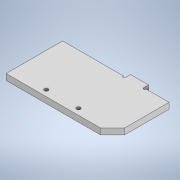
# Autodesk Inventor part: Trunk_lower_flank_frame_
Saved by Autodesk Inventor 2020.4 (Build 244396000, 396)
## iProperties
Created: 2022-01-02
Part Number: Trunk_lower_flank_frame_
Material: 一般
Document SubType Name: Modeling
Designer: Masato Kubotera
Density: 1 g/cm^3
Appearance: 既定
Author: Masato Kubotera
Autodesk Inventor part; units mm, degrees
ref_plane "YZ Plane" through (0, 0, 0) normal (1, 0, 0) x (0, 1, 0)
ref_plane "XZ Plane" through (0, 0, 0) normal (0, 1, 0) x (-1, 0, 0)
ref_plane "XY Plane" through (0, 0, 0) normal (0, 0, 1) x (1, 0, 0)
derived "Trunk_basis.ipt"
sketch "スケッチ1" plane through (0, 0, 0) normal (0, 1, 0) x (-1, 0, 0)
  line L0 (0, 24.5) -> (0, -139) construction
  circle A0 centre (5, 0) radius 10.5 construction
  line L1 (-7, 16) -> (36, 16) construction
  line L2 (36, 16) -> (36, -16) construction
  line L3 (36, -16) -> (-7, -16) construction
  line L4 (-7, -16) -> (-7, 16) construction
  line L5 (-7, 16) -> (36, -16) construction
  line L6 (36, 16) -> (-7, -16) construction
  line L7 (33, 13.5) -> (6, 13.5) construction
  line L8 (6, 13.5) -> (6, -13.5) construction
  line L9 (6, -13.5) -> (33, -13.5) construction
  line L10 (33, -13.5) -> (33, 13.5) construction
  line L11 (33, 13.5) -> (6, -13.5) construction
  line L12 (6, 13.5) -> (33, -13.5) construction
  line L13 (-7, 0) -> (36, 0) construction
  arc A1 (5, 16) -> (-7, 10.583) centre (5, 0) ccw construction
  line L14 (34.5651, -16.05) -> (5, -16.05)
  line L15 (5, 16.05) -> (34.5651, 16.05)
  line L16 (36.05, 14.5651) -> (36.05, -14.5651)
  line L17 (36.05, -16.05) -> (-7.05, 16.05) construction
  line L18 (-7.05, -16.05) -> (36.05, 16.05) construction
  arc A2 (5, 16.05) -> (-6.5314, 11.1638) centre (5, 0) ccw
  arc A3 (-6.5314, 11.1638) -> (-7.05, 9.8372) centre (-6.0721, 10.2196) ccw
  arc A4 (36.05, 14.5651) -> (34.5651, 16.05) centre (35.3075, 15.3075) ccw
  circle A5 centre (6, 13.5) radius 1.35 construction
  line L19 (19.5, 13.5) -> (19.5, -13.5) construction
  circle A6 centre (33, 13.5) radius 1.35 construction
  line L20 (-9.5, 24.5) -> (-14.5, 19.5)
  line L21 (-14.5, 19.5) -> (-14.5, -2.8299)
  line L22 (-14.5, -2.8299) -> (-28.5, -16.8299)
  line L23 (-28.5, -16.8299) -> (-28.5, -94.5)
  line L24 (86.5, -94.5) -> (86.5, -38.5827)
  line L25 (86.5, -38.5827) -> (52.05, -18.693)
  line L26 (52.05, -18.693) -> (52.05, 19.5)
  line L27 (52.05, 19.5) -> (47.05, 24.5)
  line L28 (47.05, 24.5) -> (-9.5, 24.5)
  line L29 (-18.5, -92) -> (-28.5, -102)
  line L30 (-28.5, -102) -> (-28.5, -139)
  line L31 (-28.5, -139) -> (60, -139)
  line L32 (60, -139) -> (60, -92)
  line L33 (60, -92) -> (-18.5, -92)
  line L34 (-16, -139) -> (-16, -99.5) construction
  line L35 (-16, -99.5) -> (16, -99.5) construction
  line L36 (16, -139) -> (16, -99.5) construction
  line L37 (-7.5, -139) -> (-7.5, -143)
  line L38 (-7.5, -143) -> (7.5, -143)
  line L39 (7.5, -139) -> (7.5, -143)
  arc A7 (-7.5, -139) -> (-9.6, -139) centre (-8.55, -139) ccw
  arc A8 (9.6, -139) -> (7.5, -139) centre (8.55, -139) ccw
  line L40 (-20, -139) -> (-20, -133) construction
  line L41 (-21.5, -133) -> (-18.5, -133) construction
  line L42 (-21.5, -133) -> (-21.5, -139) construction
  line L43 (-18.5, -133) -> (-18.5, -139) construction
  line L44 (-12, 22) -> (-7, 22) construction
  line L45 (-7, 22) -> (-7, -22) construction
  line L46 (-7, -22) -> (-12, -22) construction
  line L47 (-12, -22) -> (-12, 22) construction
  line L48 (-12, 22) -> (-7, -22) construction
  line L49 (-7, 22) -> (-12, -22) construction
  line L50 (-9.5, 22) -> (-9.5, -22) construction
  line L51 (-7, 0) -> (-12, 0) construction
  circle A9 centre (-9.5, 17.75) radius 1.6
  line L52 (-12, 10) -> (-9.5, 10) construction
  line L53 (-9.5, 10) -> (-9.5, -10) construction
  line L54 (-9.5, -10) -> (-12, -10) construction
  line L55 (-12, -10) -> (-12, 10) construction
  line L56 (-12, 10) -> (-9.5, -10) construction
  line L57 (-9.5, 10) -> (-12, -10) construction
  line L58 (-9.45, 10.05) -> (-12.05, 10.05)
  line L59 (-12.05, 7.95) -> (-12.05, -7.95)
  line L60 (-12.05, -10.05) -> (-9.45, -10.05)
  line L61 (-9.45, -7.95) -> (-9.45, 7.95)
  line L62 (-9.45, 10.05) -> (-12.05, -10.05) construction
  line L63 (-12.05, 10.05) -> (-9.45, -10.05) construction
  arc A10 (-12.05, 10.05) -> (-12.05, 7.95) centre (-12.05, 9) ccw
  line L64 (-10.75, 10) -> (-10.75, -10) construction
  arc A11 (-9.45, 7.95) -> (-9.45, 10.05) centre (-9.45, 9) ccw
  circle A12 centre (-9.5, -17.75) radius 1.6
  arc A13 (-12.05, -7.95) -> (-12.05, -10.05) centre (-12.05, -9) ccw
  arc A14 (-9.45, -10.05) -> (-9.45, -7.95) centre (-9.45, -9) ccw
  line L65 (36.05, 14.4) -> (44.55, 14.4) construction
  line L66 (44.55, 14.4) -> (44.55, -14.4) construction
  line L67 (36.05, -14.4) -> (44.55, -14.4) construction
  line L68 (44.5, 7.95) -> (44.5, -7.95)
  line L69 (49.55, 0) -> (44.55, 0) construction
  line L70 (44.55, 22) -> (49.55, 22) construction
  line L71 (47.1, -7.95) -> (47.1, 7.95)
  line L72 (45.8, 10) -> (45.8, -10) construction
  line L73 (47.05, 10) -> (44.55, -10) construction
  line L74 (47.05, -10) -> (44.55, -10) construction
  line L75 (47.05, 10) -> (47.05, -10) construction
  line L76 (44.55, 10) -> (47.05, -10) construction
  line L77 (44.5, -10.05) -> (47.1, -10.05)
  line L78 (44.5, 10.05) -> (47.1, -10.05) construction
  line L79 (47.1, 10.05) -> (44.5, -10.05) construction
  line L80 (49.55, -22) -> (44.55, -22) construction
  line L81 (44.55, 22) -> (49.55, -22) construction
  line L82 (49.55, 22) -> (49.55, -22) construction
  line L83 (49.55, 22) -> (44.55, -22) construction
  line L84 (47.05, 22) -> (47.05, -22) construction
  line L85 (44.55, -22) -> (44.55, 22) construction
  circle A15 centre (47.05, -17.75) radius 1.6
  arc A16 (47.1, -10.05) -> (47.1, -7.95) centre (47.1, -9) ccw
  line L86 (44.55, -10) -> (44.55, 10) construction
  arc A17 (44.5, -7.95) -> (44.5, -10.05) centre (44.5, -9) ccw
  arc A18 (44.5, 10.05) -> (44.5, 7.95) centre (44.5, 9) ccw
  arc A19 (47.1, 7.95) -> (47.1, 10.05) centre (47.1, 9) ccw
  line L87 (44.55, 10) -> (47.05, 10) construction
  line L88 (47.1, 10.05) -> (44.5, 10.05)
  circle A20 centre (47.05, 17.75) radius 1.6
  line L89 (-18.5, -104.5) -> (-28.5, -94.5)
  line L90 (-18.5, -104.5) -> (60, -104.5)
  circle A21 centre (4.848, -97) radius 1.6
  line L91 (-16, -94.5) -> (52.5, -94.5) construction
  line L92 (52.5, -94.5) -> (52.5, -99.5) construction
  line L93 (52.5, -99.5) -> (-16, -99.5) construction
  line L94 (-16, -99.5) -> (-16, -94.5) construction
  line L95 (-16, -94.5) -> (52.5, -99.5) construction
  line L96 (52.5, -94.5) -> (-16, -99.5) construction
  line L97 (-16, -97) -> (52.5, -97) construction
  line L98 (-18.5, -92) -> (-18.5, -104.5) construction
  line L99 (18.25, -99.5) -> (18.25, -94.5) construction
  circle A22 centre (31.652, -97) radius 1.6
  line L100 (-28.5, -94.5) -> (86.5, -94.5) construction
  line L101 (86.5, -94.5) -> (60, -104.5)
  circle A23 centre (5, 0) radius 16 construction
  arc A24 (-6.5314, -11.1638) -> (5, -16.05) centre (5, 0) ccw
  arc A25 (-7.05, -9.8372) -> (-6.5314, -11.1638) centre (-6.0721, -10.2196) ccw
  arc A26 (34.5651, -16.05) -> (36.05, -14.5651) centre (35.3075, -15.3075) ccw
  line L102 (-7.05, -9.8372) -> (-7.05, 9.8372)
  line L103 (20, -139) -> (20, -133) construction
  line L104 (21.5, -133) -> (21.5, -139) construction
  line L105 (18.5, -133) -> (18.5, -139) construction
  line L106 (21.5, -133) -> (18.5, -133) construction
  circle A27 centre (6, -13.5) radius 1.35
  circle A28 centre (33, -13.5) radius 1.35
  point P0 (0, 0)
  point P1 (14.5, 0)
  point P2 (19.5, 0)
  point P3 (-7.05, 10.6019)
  point P4 (19.5, 0)
  point P5 (-9.5, 0)
  point P6 (-10.75, 0)
  point P7 (45.8, 0)
  point P8 (47.05, 0)
  point P9 (18.25, -97)
  dimension "d4" = 40
  measures "d4" distance of L103.start L40.start
extrude "押し出し1" add sketch "スケッチ1" along normal blind 5 contours L89 L90 L32 L31 A8 A7 L30 L29 | L29 L33 L32 L90 L89 | L31 L39 L38 L37
sketch "スケッチ2" plane through (28.5, 0, -139) normal (0, 0, -1) x (-1, 0, 0)
  line L0 (0, 0) -> (0, 5) projected
  line L1 (0, 2.5) -> (88.5, 2.5)
  line L2 (88.5, 0) -> (88.5, 5) projected
  line L3 (28.5, 0) -> (28.5, 5)
  line L4 (21, 5) -> (36, 5) projected
  point P0 (8.5, 2.5)
  point P1 (48.5, 2.5)
  dimension "d3" = 40
  constraints: 4 end point, 3 midpoint, 1 point on line, 1 symmetric about line, 1 vertical
  measures "d3" distance of point (48.5, 2.5) point (8.5, 2.5)
hole "穴1" at (20, 2.5, -139) at (-20, 2.5, -139) direction (0, 0, 1) diameter 2.459 depth 6 tip angle 118 thread size "M3x0.5" class "6H" standard "ISO Metric profile"
equation "\"d3\" = d4"
